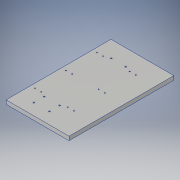
# Autodesk Inventor part: mplate
Saved by Autodesk Inventor 2019 (Build 230136000, 136)
## iProperties
Created: 2022-09-05
Part Number: mplate
Material: Aluminum 6061
Document SubType Name: Modeling
Designer: kananovicha
Density: 2.7 g/cm^3
Appearance: Aluminum - Flat
Author: kananovicha
Autodesk Inventor part; units mm, degrees
ref_plane "YZ Plane" through (0, 0, 0) normal (1, 0, 0) x (0, 1, 0)
ref_plane "XZ Plane" through (0, 0, 0) normal (0, 1, 0) x (-1, 0, 0)
ref_plane "XY Plane" through (0, 0, 0) normal (0, 0, 1) x (1, 0, 0)
sketch "Sketch1" plane through (0, 0, 0) normal (0, 0, 1) x (1, 0, 0)
  line L0 (-152.4, 9.525) -> (152.4, 9.525)
  line L1 (152.4, 9.525) -> (152.4, -9.525)
  line L2 (152.4, -9.525) -> (-152.4, -9.525)
  line L3 (-152.4, -9.525) -> (-152.4, 9.525)
  line L4 (-152.4, 9.525) -> (152.4, -9.525) construction
  line L5 (152.4, 9.525) -> (-152.4, -9.525) construction
  point P0 (0, 0)
  dimension "d0" = 304.8
  dimension "d1" = 19.05
  constraints: 12 end point, 2 midpoint, 2 parallel, 1 horizontal, 1 perpendicular
  measures "d0" distance of L1.end L2.end
  measures "d1" distance of L0.end L1.end
extrude "Extrusion1" add sketch "Sketch1" against normal blind 508
sketch "Sketch2" plane through (-152.4, 9.525, 0) normal (0, 1, 0) x (1, 0, 0)
  line L0 (0, 0) -> (0, 508) projected
  line L1 (0, 0) -> (304.8, 0) projected
  point P0 (152.4, 0)
  point P1 (78.58, 56)
  dimension "d4" = 78.58
  dimension "d5" = 56
  measures "d4" distance from line of point (78.58, 56) L0
  measures "d5" distance from line of point (78.58, 56) L1
hole "Hole1" at (-73.82, 9.525, -56) direction (0, -1, 0) diameter 6.6548 end through all
pattern_linear "Rectangular Pattern1" count 2 spacing 50 along (0, 0, -1) count 2 spacing 75 along (1, 0, 0) of "Hole1"
sketch "Sketch3" plane through (-152.4, 9.525, 0) normal (0, 1, 0) x (1, 0, 0)
  line L0 (0, 0) -> (304.8, 0) projected
  line L1 (0, 0) -> (0, 508) projected
  point P0 (152.4, 0)
  point P1 (81.08, 428.5012)
  point P2 (151.08, 428.5012)
  dimension "d25" = 428.5012
  dimension "d26" = 81.08
  dimension "d27" = 428.5012
  dimension "d28" = 70
  measures "d25" distance from line of L0 point (81.08, 428.501)
  measures "d26" distance from line of L1 point (81.08, 428.501)
  measures "d27" distance from line of point (151.08, 428.501) L0
  measures "d28" distance of point (81.08, 428.501) point (151.08, 428.501)
hole "Hole2" at (-71.32, 9.525, -428.5012) at (-1.32, 9.525, -428.5012) direction (0, -1, 0) diameter 6.6548 end through all
sketch "Sketch4" plane through (-152.4, 9.525, 0) normal (0, 1, 0) x (1, 0, 0)
  line L0 (0, 0) -> (0, 508) projected
  line L1 (0, 0) -> (304.8, 0) projected
  point P0 (152.4, 0)
  point P1 (21.873, 118.25)
  dimension "d36" = 21.873
  dimension "d37" = 118.25
  measures "d36" distance from line of point (21.873, 118.25) L0
  measures "d37" distance from line of point (21.873, 118.25) L1
hole "Hole3" at (-130.527, 9.525, -118.25) direction (0, -1, 0) diameter 4.9276 end through all
pattern_linear "Rectangular Pattern3" count 3 spacing 150 along (0, 0, -1) count 2 spacing 29.9974 along (1, 0, 0) of "Hole3"
sketch "Sketch5" plane through (-152.4, 9.525, 0) normal (0, 1, 0) x (1, 0, 0)
  line L0 (304.8, 0) -> (304.8, 508) projected
  line L1 (0, 0) -> (304.8, 0) projected
  point P0 (152.4, 0)
  point P1 (210.287, 118.25)
  dimension "d51" = 94.513
  dimension "d52" = 118.25
  measures "d51" distance from line of point (210.287, 118.25) L0
  measures "d52" distance from line of point (210.287, 118.25) L1
hole "Hole4" at (57.887, 9.525, -118.25) direction (0, -1, 0) diameter 4.9276 end through all
pattern_linear "Rectangular Pattern4" count 3 spacing 150 along (0, 0, -1) count 2 spacing 29.9974 along (-1, 0, 0) of "Hole4"
equation "\"d0\" = mp_wid"
equation "\"d1\" = mp_thick"
equation "\"d2\" = mp_len"
equation "\"d4\" = mp_mbra_holes_w_offset"
equation "\"d5\" = mp_mbra_holes_l_offset"
equation "\"d15\" = mp_mbra_holes_l_spacing"
equation "\"d18\" = mp_mbra_holes_w_spacing"
equation "\"d25\" = mp_bf_holes_l_offset"
equation "\"d26\" = mp_bf_holes_w_offset"
equation "\"d27\" = mp_bf_holes_l_offset"
equation "\"d28\" = mp_bf_holes_w_spacing"
equation "\"d36\" = mp_brm_w_offset + brm_hole_h_offset"
equation "\"d37\" = asse_brm_l_offset + brm_hole_v_offset"
equation "\"d47\" = brm_hole_v_spacing"
equation "\"d50\" = brm_hole_h_spacing"
equation "\"d51\" = mp_brm_w_offset_right + brm_hole_h_offset"
equation "\"d52\" = asse_brm_l_offset + brm_hole_v_offset"
equation "\"d62\" = brm_hole_v_spacing"
equation "\"d65\" = brm_hole_h_spacing"
equation "\"mp_wid\" = 304.8"
equation "\"mp_thick\" = 19.05"
equation "\"mp_len\" = 508"
equation "\"mp_mbra_holes_l_spacing\" = 50"
equation "\"mp_mbra_holes_w_spacing\" = 75"
equation "\"brm_hole_v_spacing\" = 150"
equation "\"brm_hole_h_spacing\" = 29.9974"
equation "\"mp_mbra_holes_w_offset\" = 78.58"
equation "\"mp_mbra_holes_l_offset\" = 56"
equation "\"mp_bf_holes_l_offset\" = 428.50116"
equation "\"mp_bf_holes_w_offset\" = 81.08"
equation "\"mp_bf_holes_w_spacing\" = 70"
equation "\"mp_brm_w_offset\" = 14.38"
equation "\"brm_hole_h_offset\" = 7.493"
equation "\"asse_brm_l_offset\" = 68.25"
equation "\"brm_hole_v_offset\" = 50"
equation "\"mp_brm_w_offset_right\" = 87.02"
body "Solid1"
